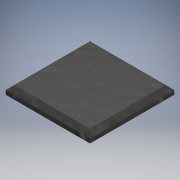
# Autodesk Inventor part: Bit Nhom 3060
Saved by Autodesk Inventor 2019 (Build 230136000, 136)
## iProperties
Created: 2019-05-17
Part Number: Bit Nhom 3060
Material: Generic
Document SubType Name: Modeling
Designer: Admin
Density: 1 g/cm^3
Appearance: Fine Textured - Black
Author: Admin
Autodesk Inventor part; units mm, degrees
ref_plane "YZ Plane" through (0, 0, 0) normal (1, 0, 0) x (0, 1, 0)
ref_plane "XZ Plane" through (0, 0, 0) normal (0, 1, 0) x (-1, 0, 0)
ref_plane "XY Plane" through (0, 0, 0) normal (0, 0, 1) x (1, 0, 0)
sketch "Sketch1" plane through (0, 0, 0) normal (0, 0, 1) x (1, 0, 0)
  line L0 (-10, -10) -> (10, -10)
  line L1 (10, -10) -> (10, 10)
  line L2 (10, 10) -> (-10, 10)
  line L3 (-10, 10) -> (-10, -10)
  line L4 (-10, -10) -> (10, 10) construction
  line L5 (10, -10) -> (-10, 10) construction
  point P0 (0, 0)
  dimension "d0" = 20
  dimension "d1" = 20
  constraints: 12 end point, 2 midpoint, 2 parallel, 1 horizontal, 1 perpendicular
  measures "d0" distance of L2.end L1.end
  measures "d1" distance of L1.end L0.end
extrude "Extrusion1" add sketch "Sketch1" along normal blind 2
chamfer "Chamfer1" distance 1 angle 45 1 edges at (0, 10, 2)
chamfer "Chamfer2" distance 1 angle 45 3 edges at (10, -0.5, 2) (-10, -0.5, 2) (0, -10, 2)
body "Solid1"
